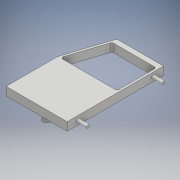
# Autodesk Inventor part: PuertaAdelante
Saved by Autodesk Inventor 2017 (Build 210142000, 142)
## iProperties
Part Number: PuertaAdelante
Material: Genérico
Document SubType Name: Modeling
Designer: Ghost
Density: 1 g/cm^3
Appearance: Valor por defecto
Author: Ghost
Autodesk Inventor part; units mm, degrees
ref_plane "YZ Plane" through (0, 0, 0) normal (1, 0, 0) x (0, 1, 0)
ref_plane "XZ Plane" through (0, 0, 0) normal (0, 1, 0) x (-1, 0, 0)
ref_plane "XY Plane" through (0, 0, 0) normal (0, 0, 1) x (1, 0, 0)
sketch "Boceto1" plane through (0, 0, 0) normal (0, 0, 1) x (1, 0, 0)
  line L0 (0, 0) -> (0, 49.6834)
  line L1 (0.0978, 50.3011) -> (13.4493, 91.4177)
  line L2 (58.8982, 92.8) -> (58.8982, 0)
  arc A0 (15.3516, 92.8) -> (13.4493, 91.4177) centre (15.3516, 90.8) ccw
  arc A1 (0.0978, 50.3011) -> (0, 49.6834) centre (2, 49.6834) ccw
  line L3 (2.9528, 52.6177) -> (13.9285, 86.4177)
  line L4 (15.8307, 87.8) -> (54.8982, 87.8)
  line L5 (56.8982, 85.8) -> (56.8982, 52)
  line L6 (54.8982, 50) -> (4.8551, 50)
  arc A2 (15.8307, 87.8) -> (13.9285, 86.4177) centre (15.8307, 85.8) ccw
  arc A3 (56.8982, 85.8) -> (54.8982, 87.8) centre (54.8982, 85.8) ccw
  arc A4 (54.8982, 50) -> (56.8982, 52) centre (54.8982, 52) ccw
  arc A5 (2.9528, 52.6177) -> (4.8551, 50) centre (4.8551, 52) ccw
  line L7 (0, 0) -> (58.8982, 0)
  line L8 (15.3516, 92.8) -> (58.8982, 92.8)
  point P0 (0, 50)
  point P1 (13.8982, 92.8)
  point P2 (2.1028, 50)
  point P3 (0.0246, 49.9961)
  dimension "d31" = 45
  dimension "d32" = 50
  dimension "d33" = 45
  dimension "d43" = 2
  dimension "d48" = 2
  dimension "d49" = 2
  dimension "d50" = 2
  dimension "d57" = 92.8
  dimension "d58" = 5
  dimension "d59" = 13.4493
  dimension "d60" = 162.01
  constraints: 18 end point, 13 point on circle, 11 tangent, 6 centre point, 5 point on line, 4 horizontal, 3 equal radius, 2 vertical, 1 horizontal alignment, 1 parallel
  measures "d31" distance of point (0, 50) point (13.898, 92.8)
  measures "d32" distance of L0.start point (0, 50)
  measures "d33" distance from line of L2 point (13.898, 92.8)
  measures "d43" radius of A0
  measures "d48" distance between parallel lines of L2 L5
  measures "d49" distance between parallel lines of L1 L3
  measures "d50" radius of A2
  measures "d57" distance of L2.start L2.end
  measures "d58" distance between parallel lines of L8 L4
  measures "d59" horizontal distance of point (0, 50) L1.end
  measures "d60" angle of L1 L0
extrude "Extrusión3" add sketch "Boceto1" against normal blind 8
sketch "Boceto2" plane through (58.8982, 0, 0) normal (1, 0, 0) x (0, 0, -1)
  circle A0 centre (4, 10) radius 1.5
  circle A1 centre (4, 82.8) radius 1.5
  line L0 (0, 0) -> (8, 0) projected
  line L1 (0, 0) -> (0, 49.6834) projected
  line L2 (0, 92.8) -> (8, 92.8) projected
  line L3 (0, 92.8) -> (0, 0) projected
  dimension "d61" = 3
  dimension "d62" = 10
  dimension "d63" = 4
  dimension "d64" = 10
  dimension "d65" = 4
  constraints: 2 centre point, 1 equal radius
  measures "d61" diameter of A0
  measures "d62" distance from line of L0 A0.centre
  measures "d63" distance from line of L1 A0.centre
  measures "d64" distance from line of L2 A1.centre
  measures "d65" distance from line of L3 A1.centre
extrude "Extrusión4" add sketch "Boceto2" along normal blind 10
sketch "Boceto3" plane through (0, 0, -8) normal (0, 0, -1) x (-1, 0, 0)
  circle A0 centre (-29.4582, 10) radius 4
  line L0 (-58.8982, 0) -> (0, 0) projected
  line L1 (-58.8982, 92.8) -> (-58.8982, 0) projected
  dimension "d68" = 10
  dimension "d69" = 29.44
  dimension "d72" = 8
  constraints: 1 centre point
  measures "d68" distance from line of L0 A0.centre
  measures "d69" distance from line of A0.centre L1
  measures "d72" diameter of A0
extrude "Extrusión5" add sketch "Boceto3" along normal blind 10
